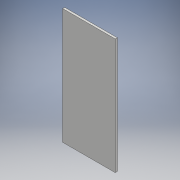
# Autodesk Inventor part: 洞洞板
Saved by Autodesk Inventor 2018 (Build 220112000, 112)
## iProperties
Created: 2020-11-25
Part Number: 洞洞板
Material: 常规
Document SubType Name: Modeling
Designer: OHHHHHHHHHH
Density: 1 g/cm^3
Appearance: 默认
Author: OHHHHHHHHHH
Autodesk Inventor part; units mm, degrees
ref_plane "YZ Plane" through (0, 0, 0) normal (1, 0, 0) x (0, 1, 0)
ref_plane "XZ Plane" through (0, 0, 0) normal (0, 1, 0) x (-1, 0, 0)
ref_plane "XY Plane" through (0, 0, 0) normal (0, 0, 1) x (1, 0, 0)
sketch "草图1" plane through (0, 0, 0) normal (0, 1, 0) x (-1, 0, 0)
  line L0 (0, 0) -> (25, 0)
  line L1 (25, 0) -> (25, -55)
  line L2 (25, -55) -> (0, -55)
  line L3 (0, -55) -> (0, 0)
  dimension "d0" = 25
  dimension "d1" = 55
  constraints: 8 end point, 2 parallel, 1 horizontal, 1 perpendicular
  measures "d0" distance of L0.start L0.end
  measures "d1" distance of L2.end L0.start
extrude "拉伸1" add sketch "草图1" along normal blind 1
sketch "草图2" plane through (0, 1, 0) normal (0, 1, 0) x (1, 0, 0)
  line L0 (-18.2717, 15.2493) -> (-5.6968, 15.2493) construction
  line L1 (-5.6968, 15.2493) -> (-5.6968, 11.401) construction
  line L2 (-5.6968, 11.401) -> (-18.2717, 11.401) construction
  line L3 (-18.2717, 11.401) -> (-18.2717, 15.2493) construction
  constraints: 2 other
